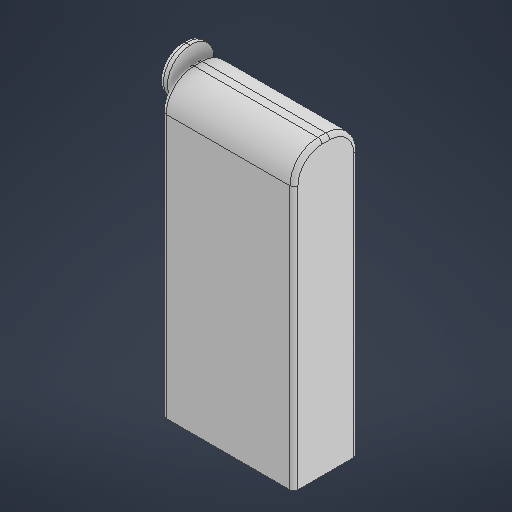
# Autodesk Inventor part: Battery
Saved by Autodesk Inventor 2027 (Build 310192000, 192)
## iProperties
Created: 2026-04-23
Part Number: Battery
Material: Generic
Document SubType Name: Modeling
Designer: angel
Density: 1 g/cm^3
Appearance: Default
Author: angel
Autodesk Inventor part; units mm, degrees
ref_plane "YZ Plane" through (0, 0, 0) normal (1, 0, 0) x (0, 1, 0)
ref_plane "XZ Plane" through (0, 0, 0) normal (0, 1, 0) x (-1, 0, 0)
ref_plane "XY Plane" through (0, 0, 0) normal (0, 0, 1) x (1, 0, 0)
sketch "Sketch1" plane through (0, 0, 0) normal (0, 0, 1) x (1, 0, 0)
  line L0 (0, 0) -> (33, 0)
  line L1 (33, 0) -> (33, 73)
  line L2 (33, 73) -> (0, 73)
  line L3 (0, 73) -> (0, 0)
  dimension "d0" = 33
  dimension "d1" = 73
  constraints: 8 end point, 2 parallel, 1 horizontal, 1 perpendicular
  measures "d0" distance of L2.end L1.end
  measures "d1" distance between parallel lines of L0 L2
extrude "Extrusion1" add sketch "Sketch1" along normal blind 16
fillet "Fillet1" radius 7 2 edges at (16.5, 73, 16) (16.5, 73, 0)
fillet "Fillet2" radius 1 10 edges at (0, 70.9497, 13.9497) (0, 73, 8) (0, 70.9497, 2.0503) (0, 33, 0) (0, 33, 16) (33, 70.9497, 13.9497) (33, 73, 8) (33, 70.9497, 2.0503) (33, 33, 0) (33, 33, 16)
sketch "Sketch2" plane through (0, 0, 1) normal (-1, 0, 0) x (0, 0, 1)
  line L0 (14, 66) -> (15, 66) construction
  line L1 (14, 66) -> (14, 68.5) construction
  arc A0 (14, 66) -> (8, 72) centre (8, 66) ccw construction
  line L2 (14, 68.5) -> (-0.5383, 68.5) construction
  arc A1 (6, 73) -> (-1, 66) centre (6, 66) ccw construction
  line L3 (-1, 66) -> (3, 66) construction
  line L4 (3, 66) -> (3, 68.5) construction
  line L5 (14, 68.5) -> (12, 68.5) construction
  arc A2 (3, 68.5) -> (13, 68.5) centre (8, 86.046) ccw
  arc A3 (15, 66) -> (8, 73) centre (8, 66) ccw projected
  line L6 (8, 72) -> (8, 73) construction
  line L7 (8, 73) -> (8, 77) construction
  arc A4 (8, 77) -> (3, 68.5) centre (7.5155, 71.5644) ccw
  arc A5 (13, 68.5) -> (8, 77) centre (7.9605, 71.2562) ccw
  point P0 (-1, 0)
  dimension "d6" = 2.5
  dimension "d7" = 4
  dimension "d8" = 2
  dimension "d9" = 4
  dimension "d10" = 18.2445
  dimension "d11" = 5.7439
  dimension "d12" = 5.4571
  constraints: 12 end point, 7 point on circle, 3 centre point, 2 horizontal, 2 point on line, 2 vertical, 1 midpoint, 1 perpendicular, 1 tangent
  measures "d6" distance of L0.start L1.end
  measures "d7" distance of L3.start L3.end
  measures "d8" distance of L1.end L5.end
  measures "d9" distance of L6.end L7.end
  measures "d10" radius of A2
  measures "d11" radius of A5
  measures "d12" radius of A4
extrude "Extrusion2" add sketch "Sketch2" along normal blind 2
fillet "Fillet3" radius 1 3 edges at (-2, 74.1685, 13.9114) (-2, 67.8015, 9) (-2, 74.3313, 3.8118)
body "Solid1"
